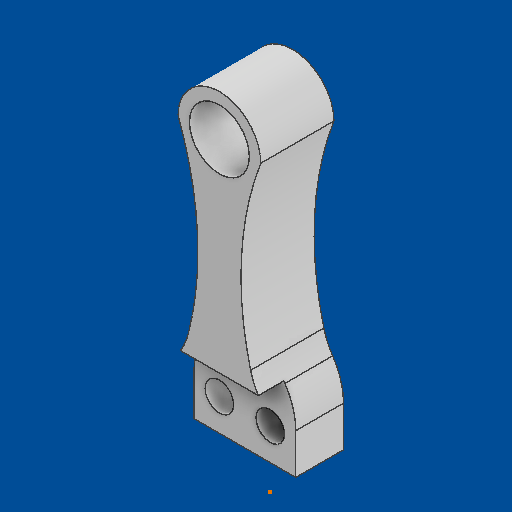
# Autodesk Inventor part: pawn
Saved by Autodesk Inventor 2026.2 (Build 302298000, 298)
## iProperties
Created: 2026-01-15
Part Number: pawn
Material: Generic
Document SubType Name: Modeling
Designer: Thoma
Density: 1 g/cm^3
Appearance: Default
Author: Thoma
Autodesk Inventor part; units mm, degrees
ref_plane "YZ Plane" through (0, 0, 0) normal (1, 0, 0) x (0, 1, 0)
ref_plane "XZ Plane" through (0, 0, 0) normal (0, 1, 0) x (-1, 0, 0)
ref_plane "XY Plane" through (0, 0, 0) normal (0, 0, 1) x (1, 0, 0)
sketch "Sketch1" plane through (0, 0, 0) normal (0, 1, 0) x (-1, 0, 0)
  line L0 (0, 0) -> (16, 0)
  line L1 (16, 0) -> (16, -12.3)
  line L2 (16, -12.3) -> (0, -12.3)
  line L3 (0, -12.3) -> (0, 0)
  dimension "d0" = 16
  dimension "d1" = 12.3
  constraints: 8 end point, 2 parallel, 1 horizontal, 1 perpendicular
  measures "d0" distance of L1.end L2.end
  measures "d1" distance of L0.end L1.end
extrude "Extrusion1" add sketch "Sketch1" along normal blind 10
sketch "Sketch2" plane through (0, 10, 0) normal (0, 1, 0) x (1, 0, 0)
  line L0 (-16, 0) -> (0, 0) projected
  line L1 (-8, 0) -> (-8, 12.3)
  line L2 (0, 12.3) -> (-16, 12.3) projected
  line L3 (-14.5, 0) -> (-14.5, 12.3)
  line L4 (-1.5, 0) -> (-1.5, 12.3)
  dimension "d4" = 6.5
  dimension "d5" = 6.5
  constraints: 6 end point, 4 point on line, 2 midpoint, 2 perpendicular
  measures "d4" distance between parallel lines of L1 L3
  measures "d5" distance between parallel lines of L1 L4
extrude "Extrusion2" add sketch "Sketch2" along normal blind 40.5
sketch "Sketch3" plane through (-16, 0, 0) normal (0, 0, 1) x (1, 0, 0)
  line L0 (14.5, 50.5) -> (1.5, 50.5) projected
  line L1 (8, 50.5) -> (8, 0)
  line L2 (0, 0) -> (16, 0) projected
  circle A0 centre (8, 44) radius 4.5
  line L3 (1.5, 50.5) -> (14.5, 50.5) projected
  circle A1 centre (8, 44) radius 6.5
  line L4 (14.5, 10) -> (14.5, 50.5) projected
  line L5 (14.5, 30.25) -> (1.5, 30.25)
  line L6 (1.5, 10) -> (1.5, 50.5) projected
  line L7 (8, 30.25) -> (11.5, 30.25)
  arc A2 (14.5, 44) -> (14.5, 10) centre (59.4062, 27) ccw
  line L8 (8, 30.25) -> (4.5, 30.25)
  arc A3 (1.5, 10) -> (1.5, 44) centre (-43.4062, 27) ccw
  dimension "d8" = 6.5
  dimension "d9" = 9
  dimension "d10" = 13
  dimension "d11" = 3.5
  dimension "d12" = 3.5
  constraints: 8 end point, 8 point on circle, 6 midpoint, 5 point on line, 4 centre point, 1 coincident, 1 tangent
  measures "d8" distance of A0.centre point (8, 50.5)
  measures "d9" diameter of A0
  measures "d10" diameter of A1
  measures "d11" distance of L7.end L7.start
  measures "d12" distance of L7.start L8.end
extrude "Extrusion3" cut sketch "Sketch3" against normal blind 13.5 contours L4 A1 L0 | A1 L6 L0 | L4 L5 A2 A1 | A1 A2 | A3 A1 | A1 A3 L5 L6 | L4 A2 L5 | L5 A3 L6
fillet "Fillet1" radius 10 4 edges at (0, 10, -6.15) (-1.5, 10, -6.15) (-14.5, 10, -6.15) (-16, 10, -6.15)
sketch "Sketch4" plane through (-16, 0, 0) normal (0, 0, 1) x (1, 0, 0)
  arc A0 (14.5, 44) -> (1.5, 44) centre (8, 44) ccw projected
  circle A1 centre (8, 44) radius 4.5
  point P0 (16, 0)
  dimension "d16" = 9
  constraints: 1 centre point, 1 coincident
  measures "d16" diameter of A1
extrude "Extrusion4" cut sketch "Sketch4" against normal blind 8.23
sketch "Sketch5" plane through (0, 0, 0) normal (0, -1, 0) x (1, 0, 0)
  point P0 (0, 0)
sketch "Sketch7" plane through (-16, 0, 0) normal (0, 0, 1) x (1, 0, 0)
  line L0 (16, 0) -> (0, 0) projected
  line L1 (0, 0) -> (16, 0)
  line L2 (16, 0) -> (16, 10)
  line L3 (16, 10) -> (0, 10)
  line L4 (0, 10) -> (0, 0)
  line L5 (0, 5) -> (16, 5)
  line L6 (8, 10) -> (8, 0)
  circle A0 centre (4, 5) radius 1
  circle A1 centre (12, 5) radius 1
  constraints: 12 end point, 4 midpoint, 2 centre point, 2 parallel, 2 point on line, 1 horizontal, 1 perpendicular
extrude "Extrusion6" cut sketch "Sketch7" against normal blind 12.3 contours A1 L5 | L5 A1 | A0 L5 | L5 A0
sketch "Sketch8" plane through (-16, 0, 0) normal (0, 0, 1) x (1, 0, 0)
  circle A0 centre (4, 5) radius 1 projected
  circle A1 centre (4, 5) radius 2.25
  circle A2 centre (12, 5) radius 1 projected
  circle A3 centre (12, 5) radius 2.25
  point P0 (16, 0)
  dimension "d24" = 4.5
  dimension "d25" = 4.5
  constraints: 2 centre point, 2 coincident
  measures "d24" diameter of A1
  measures "d25" diameter of A3
extrude "Extrusion7" cut sketch "Sketch8" against normal blind 12.5
thicken "Thicken1" operation add thickness 0.8 both sides no extend neighbours yes toward (0, 0, 1) faces at (-6.5237, 41.6451, -12.3)
sketch "Sketch10" plane through (-16, 0, 0) normal (0, 0, 1) x (1, 0, 0)
  line L0 (0, 0) -> (16, 0)
  line L1 (16, 0) -> (16, 12)
  line L2 (16, 12) -> (0, 12)
  line L3 (0, 12) -> (0, 0)
  dimension "d30" = 12
  constraints: 8 end point, 2 parallel, 1 horizontal, 1 perpendicular
  measures "d30" distance of L0.end L1.end
extrude "Extrusion8" cut sketch "Sketch10" against normal blind 4
thicken "Thicken2" operation cut thickness 0.2 both sides no extend neighbours no toward (0, 1, 0) faces at (-10.0843, 12, -1.3333)
thicken "Thicken3" operation cut thickness 0.2 both sides no extend neighbours no toward (0.9967573, -0.0804666, 0) faces at (-3.5146, 43.6379, -5.4867)
body "Solid1"
